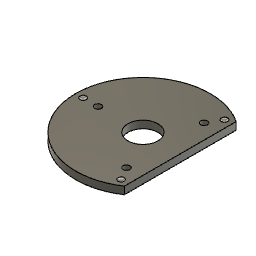
coupling assembly v2 (Autodesk Fusion 360 archive; units mm, degrees)
design "coupling bottom plate"
Autodesk Fusion 360 part; units mm, degrees
note: some values were not read from the file. Set by a fixed rule: the direction of a hole.
sketch "Sketch1" plane through (0, 0, 0) normal (0, 1, 0) x (1, 0, 0)
  circle A0 centre (0, 0) radius 50
  circle A1 centre (0, 0) radius 30 construction
  circle A2 centre (0, 0) radius 10
  circle A3 centre (0, 0) radius 45
  circle A4 centre (0, 0) radius 40 construction
  line L0 (25, -37.4166) -> (25, 37.4166)
  point P0 (-30, 0)
  point P1 (15, -25.9808)
  point P2 (15, 25.9808)
  point P3 (-40, 0)
  point P4 (20, -34.641)
  point P5 (20, 34.641)
  dimension "d1" = 100
  dimension "d2" = 60
  dimension "d3" = 20
  dimension "d4" = -5
  dimension "d6" = 360
  dimension "d14" = 80
  dimension "d18" = 5
  constraint coincident A0.centre A1.centre
  constraint concentric A1 A2
  constraint coincident A1 P0
  constraint horizontal A0.centre P0
  constraint concentric A2 A4
  constraint coincident A4 P3
  constraint horizontal A0.centre P3
  constraint coincident A3 L0.start
  constraint coincident A3 L0.end
  constraint vertical L0
  measures "d1" diameter of A0
  measures "d2" diameter of A1
  measures "d3" diameter of A2
  measures "d14" diameter of A4
  measures "d18" distance of P5 L0
extrude "Extrude1" add sketch "Sketch1" along normal blind 5 contours A3 L0 picked at (20, 0)
hole "Hole1" at (15, 0, 25.9808) at (15, 0, -25.9808) at (-30, 0, 0) direction (0, 1, 0) diameter 4.5 depth 7 tip angle 118
hole "Hole2" at (-40, 0, 0) at (20, 0, 34.641) at (20, 0, -34.641) direction (0, 1, 0) diameter 4.234 depth 25 tip angle 118
thread "Thread2" "ISO Metric profile 5.0 M5x0.8 6H"
